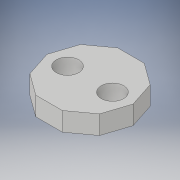
# Autodesk Inventor part: Probe P1
Saved by Autodesk Inventor 2019 (Build 230136000, 136)
## iProperties
Created: 2019-07-29
Part Number: Probe P1
Material: Generic
Document SubType Name: Modeling
Designer: azriel
Density: 1 g/cm^3
Appearance: Default
Author: azriel
Autodesk Inventor part; units mm, degrees
ref_plane "YZ Plane" through (0, 0, 0) normal (1, 0, 0) x (0, 1, 0)
ref_plane "XZ Plane" through (0, 0, 0) normal (0, 1, 0) x (-1, 0, 0)
ref_plane "XY Plane" through (0, 0, 0) normal (0, 0, 1) x (1, 0, 0)
sketch "Sketch1" plane through (0, 0, 0) normal (0, 1, 0) x (-1, 0, 0)
  circle A0 centre (0, 0) radius 13
  line L0 (-11.5, 0) -> (-9.3037, 6.7595)
  line L1 (-9.3037, 6.7595) -> (-3.5537, 10.9371)
  line L2 (-3.5537, 10.9371) -> (3.5537, 10.9371)
  line L3 (3.5537, 10.9371) -> (9.3037, 6.7595)
  line L4 (9.3037, 6.7595) -> (11.5, 0)
  line L5 (11.5, 0) -> (9.3037, -6.7595)
  line L6 (9.3037, -6.7595) -> (3.5537, -10.9371)
  line L7 (3.5537, -10.9371) -> (-3.5537, -10.9371)
  line L8 (-3.5537, -10.9371) -> (-9.3037, -6.7595)
  line L9 (-9.3037, -6.7595) -> (-11.5, 0)
  circle A1 centre (-6, 0) radius 3
  circle A2 centre (6, 0) radius 3
  dimension "d0" = 26
  dimension "d10" = 6
  dimension "d11" = 6
  constraints: 20 end point, 3 centre point, 1 coincident
  measures "d0" diameter of A0
  measures "d10" diameter of A1
  measures "d11" diameter of A2
extrude "Extrusion1" add sketch "Sketch1" against normal blind 5 contours L0 L1 L2 L3 L4 L5 L6 L7 L8 L9
body "Solid1"
